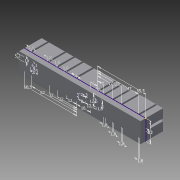
# Autodesk Inventor part: Distance_test_rig
Saved by Autodesk Inventor 2015 (Build 190159000, 159)
## iProperties
Created: 2015-05-18
Part Number: Distance_test_rig
Material: Generic
Document SubType Name: Modeling
Designer: Openlab
Density: 1 g/cm^3
Appearance: Default
Author: Openlab
Autodesk Inventor part; units mm, degrees
ref_plane "YZ Plane" through (0, 0, 0) normal (1, 0, 0) x (0, 1, 0)
ref_plane "XZ Plane" through (0, 0, 0) normal (0, 1, 0) x (-1, 0, 0)
ref_plane "XY Plane" through (0, 0, 0) normal (0, 0, 1) x (1, 0, 0)
sketch "Sketch1" plane through (0, 0, 0) normal (0, 1, 0) x (-1, 0, 0)
  line L0 (69.75, -5.25) -> (57.25, -5.25)
  line L1 (57.25, -5.25) -> (57.25, -17.75)
  line L2 (57.25, -17.75) -> (69.75, -17.75)
  line L3 (69.75, -17.75) -> (69.75, -5.25)
  line L4 (140, 0) -> (0, 0)
  line L5 (0, 0) -> (0, -23)
  line L6 (0, -23) -> (140, -23)
  line L7 (140, -23) -> (140, 0)
  line L8 (77.3838, -11.5) -> (49.3838, -11.5) construction
  line L9 (63.5, -2.25) -> (63.5, -23.25) construction
  line L10 (81.5, -8.9) -> (140, -8.9)
  line L11 (140, -14.1) -> (81.5, -14.1)
  line L12 (48.5, -23) -> (48.5, 0)
  line L13 (46.7, 0) -> (46.7, -23)
  line L14 (38.5, 0) -> (38.5, -23)
  line L15 (36.7, 0) -> (36.7, -23)
  line L16 (28.5, 0) -> (28.5, -23)
  line L17 (26.7, 0) -> (26.7, -23)
  line L18 (8.5, 0) -> (8.5, -23)
  line L19 (6.7, -23) -> (6.7, 0)
  line L20 (52, -10) -> (0, -10)
  line L21 (52, -13) -> (0, -13)
  line L22 (91.5, -14.55) -> (90, -14.55)
  line L23 (90, -14.55) -> (90, -8.45)
  line L24 (90, -8.45) -> (91.5, -8.45)
  line L25 (101.5, -14.55) -> (100, -14.55)
  line L26 (100, -14.55) -> (100, -8.45)
  line L27 (100, -8.45) -> (101.5, -8.45)
  line L28 (111.5, -14.55) -> (110, -14.55)
  line L29 (110, -14.55) -> (110, -8.45)
  line L30 (110, -8.45) -> (111.5, -8.45)
  line L31 (131.5, -14.55) -> (130, -14.55)
  line L32 (130, -14.55) -> (130, -8.45)
  line L33 (130, -8.45) -> (131.5, -8.45)
  line L34 (79.5, 0) -> (79.5, -23)
  line L35 (81.5, -23) -> (81.5, 0)
  line L36 (55.5, 0) -> (55.5, -23)
  line L37 (79.5, -13) -> (69.75, -13)
  line L38 (69.75, -10) -> (79.5, -10)
  line L39 (57.25, -13) -> (55.5, -13)
  line L40 (55.5, -10) -> (57.25, -10)
  line L41 (53.5, -15.5) -> (52, -15.5)
  line L42 (52, -15.5) -> (52, -7.5)
  line L43 (52, -7.5) -> (53.5, -7.5)
  line L44 (53.5, -23) -> (53.5, -15.5)
  line L45 (53.5, -7.5) -> (53.5, 0)
  line L46 (131.5, -17.5) -> (129.5, -17.5)
  line L47 (129.5, -17.5) -> (129.5, -15.5)
  line L48 (129.5, -15.5) -> (131.5, -15.5)
  line L49 (131.5, -7.5) -> (129.5, -7.5)
  line L50 (129.5, -7.5) -> (129.5, -5.5)
  line L51 (129.5, -5.5) -> (131.5, -5.5)
  line L52 (137, -16.5) -> (85, -16.5) construction
  line L53 (137, -6.5) -> (84.6621, -6.5) construction
  line L54 (133.3, -17.5) -> (135.3, -17.5)
  line L55 (135.3, -17.5) -> (135.3, -15.5)
  line L56 (135.3, -15.5) -> (133.3, -15.5)
  line L57 (133.3, -7.5) -> (135.3, -7.5)
  line L58 (135.3, -7.5) -> (135.3, -5.5)
  line L59 (135.3, -5.5) -> (133.3, -5.5)
  line L60 (133.3, -23) -> (133.3, -17.5)
  line L61 (131.5, -17.5) -> (131.5, -23)
  line L62 (133.3, -15.5) -> (133.3, -7.5)
  line L63 (133.3, -5.5) -> (133.3, 0)
  line L64 (131.5, 0) -> (131.5, -5.5)
  line L65 (131.5, -7.5) -> (131.5, -15.5)
  line L66 (111.5, -15.5) -> (109.5, -15.5)
  line L67 (109.5, -15.5) -> (109.5, -17.5)
  line L68 (115.3, -17.5) -> (115.3, -15.5)
  line L69 (115.3, -15.5) -> (113.3, -15.5)
  line L70 (113.3, -5.5) -> (115.3, -5.5)
  line L71 (115.3, -5.5) -> (115.3, -7.5)
  line L72 (115.3, -7.5) -> (113.3, -7.5)
  line L73 (109.5, -7.5) -> (109.5, -5.5)
  line L74 (109.5, -7.5) -> (111.5, -7.5)
  line L75 (109.5, -5.5) -> (111.5, -5.5)
  line L76 (109.5, -17.5) -> (111.5, -17.5)
  line L77 (113.3, -17.5) -> (115.3, -17.5)
  line L78 (113.3, -17.5) -> (113.3, -23)
  line L79 (111.5, -17.5) -> (111.5, -23)
  line L80 (113.3, 0) -> (113.3, -5.5)
  line L81 (113.3, -7.5) -> (113.3, -15.5)
  line L82 (111.5, 0) -> (111.5, -5.5)
  line L83 (111.5, -7.5) -> (111.5, -15.5)
  line L84 (99.5, -17.5) -> (99.5, -15.5)
  line L85 (105.3, -15.5) -> (105.3, -17.5)
  line L86 (105.3, -17.5) -> (103.3, -17.5)
  line L87 (101.5, -17.5) -> (99.5, -17.5)
  line L88 (99.5, -15.5) -> (101.5, -15.5)
  line L89 (103.3, -15.5) -> (105.3, -15.5)
  line L90 (103.3, -7.5) -> (105.3, -7.5)
  line L91 (105.3, -7.5) -> (105.3, -5.5)
  line L92 (105.3, -5.5) -> (103.3, -5.5)
  line L93 (101.5, -7.5) -> (99.5, -7.5)
  line L94 (99.5, -7.5) -> (99.5, -5.5)
  line L95 (99.5, -5.5) -> (101.5, -5.5)
  line L96 (103.3, -23) -> (103.3, -17.5)
  line L97 (101.5, -17.5) -> (101.5, -23)
  line L98 (103.3, -15.5) -> (103.3, -7.5)
  line L99 (103.3, -5.5) -> (103.3, 0)
  line L100 (101.5, 0) -> (101.5, -5.5)
  line L101 (101.5, -7.5) -> (101.5, -15.5)
  line L102 (91.5, -15.5) -> (89.5, -15.5)
  line L103 (89.5, -15.5) -> (89.5, -17.5)
  line L104 (89.5, -17.5) -> (91.5, -17.5)
  line L105 (93.3, -17.5) -> (95.3, -17.5)
  line L106 (95.3, -17.5) -> (95.3, -15.5)
  line L107 (95.3, -15.5) -> (93.3, -15.5)
  line L108 (93.3, -7.5) -> (95.3, -7.5)
  line L109 (95.3, -7.5) -> (95.3, -5.5)
  line L110 (95.3, -5.5) -> (93.3, -5.5)
  line L111 (91.5, -5.5) -> (89.5, -5.5)
  line L112 (89.5, -5.5) -> (89.5, -7.5)
  line L113 (91.5, -7.5) -> (89.5, -7.5)
  line L114 (93.3, -23) -> (93.3, -17.5)
  line L115 (91.5, -17.5) -> (91.5, -23)
  line L116 (93.3, -15.5) -> (93.3, -7.5)
  line L117 (93.3, -5.5) -> (93.3, 0)
  line L118 (91.5, 0) -> (91.5, -5.5)
  line L119 (91.5, -7.5) -> (91.5, -15.5)
  line L120 (69.75, -17.75) -> (77.75, -17.75)
  line L121 (77.75, -17.75) -> (77.75, -14.75)
  line L122 (77.75, -14.75) -> (69.75, -14.75)
  line L123 (69.75, -8.25) -> (77.75, -8.25)
  line L124 (77.75, -8.25) -> (77.75, -5.25)
  line L125 (77.75, -5.25) -> (69.75, -5.25)
  line L126 (72.75, -17.75) -> (72.75, -14.75)
  line L127 (74.75, -17.75) -> (74.75, -14.75)
  line L128 (74.75, -8.25) -> (74.75, -5.25)
  line L129 (72.75, -8.25) -> (72.75, -5.25)
  point P0 (133.3, -8.9)
  point P1 (133.3, -14.1)
  point P2 (131.5, -8.9)
  point P3 (131.5, -14.1)
  point P4 (113.3, -8.9)
  point P5 (111.5, -8.9)
  point P6 (113.3, -14.1)
  point P7 (111.5, -14.1)
  point P8 (103.3, -8.9)
  point P9 (101.5, -8.9)
  point P10 (103.3, -14.1)
  point P11 (101.5, -14.1)
  point P12 (93.3, -8.9)
  point P13 (91.5, -8.9)
  point P14 (93.3, -14.1)
  point P15 (91.5, -14.1)
  point P16 (48.5, -10)
  point P17 (46.7, -10)
  point P18 (48.5, -13)
  point P19 (46.7, -13)
  point P20 (38.5, -13)
  point P21 (36.7, -13)
  point P22 (36.7, -10)
  point P23 (38.5, -10)
  point P24 (28.5, -10)
  point P25 (26.7, -10)
  point P26 (26.7, -13)
  point P27 (28.5, -13)
  point P28 (8.5, -13)
  point P29 (6.7, -13)
  point P30 (6.7, -10)
  point P31 (8.5, -10)
  point P32 (63.5, -11.5)
  point P33 (90, -14.1)
  point P34 (90, -8.9)
  point P35 (130, -14.1)
  point P36 (130, -8.9)
  point P37 (110, -14.1)
  point P38 (110, -8.9)
  point P39 (100, -8.9)
  point P40 (100, -14.1)
  dimension "d12" = 5.2
  dimension "d25" = 3
  dimension "d0" = 12.5
  dimension "d1" = 12.5
  dimension "d3" = 23
  dimension "d18" = 1.8
  dimension "d20" = 1.8
  dimension "d22" = 1.8
  dimension "d24" = 1.8
  dimension "d36" = 6.1
  dimension "d37" = 1.5
  dimension "d43" = 2
  dimension "d62" = 3
  dimension "d63" = 3
  dimension "d70" = 60.5
  dimension "d71" = 7
  dimension "d72" = 17
  dimension "d73" = 27
  dimension "d74" = 47
  dimension "d75" = 55.5
  dimension "d91" = 8
  dimension "d92" = 1.5
  dimension "d93" = 2
  dimension "d94" = 2
  dimension "d95" = 2
  dimension "d96" = 10
  dimension "d97" = 1.8
  dimension "d98" = 52
  dimension "d99" = 1.8
  dimension "d100" = 32
  dimension "d101" = 1.8
  dimension "d102" = 22
  dimension "d103" = 1.8
  dimension "d104" = 12
  dimension "d105" = 8
  dimension "d106" = 8
  dimension "d107" = 3
  dimension "d108" = 2
  dimension "d109" = 3
  dimension "d110" = 16
  constraints: 248 end point, 113 point on line, 72 perpendicular, 44 vertical, 26 collinear, 20 equal length, 19 horizontal, 8 parallel, 1 coincident, 115 other
  measures "d0" distance of L2.end L1.end
  measures "d1" distance of L0.end L1.end
  measures "d3" distance of L5.end L5.start
  measures "d18" distance between parallel lines of L13 L12
  measures "d20" distance between parallel lines of L15 L14
  measures "d22" distance between parallel lines of L17 L16
  measures "d24" distance between parallel lines of L19 L18
  measures "d36" distance of L31.end L32.end
  measures "d37" distance of L31.start L31.end
  measures "d43" distance between parallel lines of L35 L34
  measures "d62" distance between parallel lines of L38 L37
  measures "d63" distance between parallel lines of L40 L39
  measures "d70" distance between parallel lines of L7 L34
  measures "d71" distance between parallel lines of L12 L36
  measures "d72" distance between parallel lines of L14 L36
  measures "d73" distance between parallel lines of L16 L36
  measures "d74" distance between parallel lines of L18 L36
  measures "d75" distance between parallel lines of L5 L36
  measures "d91" distance of L41.end L42.end
  measures "d92" distance of L41.start L41.end
  measures "d93" distance between parallel lines of L45 L36
  measures "d94" distance of L46.end L47.end
  measures "d95" distance of L46.start L46.end
  measures "d96" distance between parallel lines of L53 L52
  measures "d97" distance between parallel lines of L64 L63
  measures "d98" distance between parallel lines of L34 L61
  measures "d99" distance between parallel lines of L82 L80
  measures "d100" distance between parallel lines of L79 L34
  measures "d101" distance between parallel lines of L100 L99
  measures "d102" distance between parallel lines of L34 L97
  measures "d103" distance between parallel lines of L118 L117
  measures "d104" distance between parallel lines of L115 L34
  measures "d105" distance between parallel lines of L36 L9
  measures "d106" distance of L2.end L120.end
  measures "d107" distance between parallel lines of L126 L3
  measures "d108" distance between parallel lines of L126 L127
  measures "d109" distance of L120.end L121.end
  measures "d110" distance between parallel lines of L34 L9
extrude "Extrusion10" add sketch "Sketch1" against normal blind 6
extrude "Extrusion12" add sketch "Sketch1" along normal blind 5 contours L0 L1 L40 L36 L4 L34 L38 L3 L123 L124 L125 | L1 L39 L36 L40 | L38 L34 L37 L3 | L1 L2 L120 L121 L122 L3 L37 L34 L6 L36 L39 | L45 L43 L42 L20 L12 L4 | L4 L118 L111 L112 L113 L119 L24 L23 L10 L35 | L6 L12 L21 L42 L41 L44 | L35 L11 L23 L22 L119 L102 L103 L104 L115 L6 | L10 L23 L11 L35 | L13 L20 L14 L4 | L20 L42 L21 L12 | L4 L100 L95 L94 L93 L101 L27 L26 L10 L116 L108 L109 L110 L117 | L6 L14 L21 L13 | L13 L21 L14 L20 | L114 L105 L106 L107 L116 L11 L26 L25 L101 L88 L84 L87 L97 L6 | L15 L20 L16 L4 | L4 L82 L75 L73 L74 L83 L30 L29 L10 L98 L90 L91 L92 L99 | L10 L26 L11 L116 | L6 L16 L21 L15 | L15 L21 L16 L20 | L96 L86 L85 L89 L98 L11 L29 L28 L83 L66 L67 L76 L79 L6 | L17 L20 L18 L4 | L4 L64 L51 L50 L49 L65 L33 L32 L10 L81 L72 L71 L70 L80 | L6 L18 L21 L17 | L17 L21 L18 L20 | L78 L77 L68 L69 L81 L11 L32 L31 L65 L48 L47 L46 L61 L6 | L10 L29 L11 L98 | L19 L20 L5 L4 | L4 L7 L10 L62 L57 L58 L59 L63 | L6 L5 L21 L19 | L19 L21 L5 L20 | L60 L54 L55 L56 L62 L11 L7 L6 | L7 L11 L62 L10 | L10 L32 L11 L81
extrude "Extrusion13" add sketch "Sketch1" along normal blind 20 contours L0 L1 L40 L36 L4 L34 L38 L3 L123 L124 L125 | L1 L2 L120 L121 L122 L3 L37 L34 L6 L36 L39 | L45 L43 L42 L20 L12 L4 | L4 L118 L111 L112 L113 L119 L24 L23 L10 L35 | L6 L12 L21 L42 L41 L44 | L35 L11 L23 L22 L119 L102 L103 L104 L115 L6 | L13 L20 L14 L4 | L4 L100 L95 L94 L93 L101 L27 L26 L10 L116 L108 L109 L110 L117 | L6 L14 L21 L13 | L114 L105 L106 L107 L116 L11 L26 L25 L101 L88 L84 L87 L97 L6 | L15 L20 L16 L4 | L4 L82 L75 L73 L74 L83 L30 L29 L10 L98 L90 L91 L92 L99 | L6 L16 L21 L15 | L96 L86 L85 L89 L98 L11 L29 L28 L83 L66 L67 L76 L79 L6 | L17 L20 L18 L4 | L4 L64 L51 L50 L49 L65 L33 L32 L10 L81 L72 L71 L70 L80 | L6 L18 L21 L17 | L78 L77 L68 L69 L81 L11 L32 L31 L65 L48 L47 L46 L61 L6 | L19 L20 L5 L4 | L4 L7 L10 L62 L57 L58 L59 L63 | L6 L5 L21 L19 | L60 L54 L55 L56 L62 L11 L7 L6
extrude "Extrusion14" add sketch "Sketch1" along normal blind 2.5 contours L3 L2 L1 L0 | L125 L129 L123 L3 | L38 L34 L37 L3 | L125 L124 L123 L128 | L1 L2 L120 L121 L122 L3 L37 L34 L6 L36 L39 | L122 L126 L120 L3 | L122 L121 L120 L127
extrude "Extrusion15" add sketch "Sketch1" along normal blind 11.5 contours L125 L128 L123 L129 | L122 L127 L120 L126
body "Solid3"
